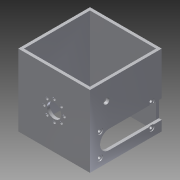
# Autodesk Inventor part: 06
Saved by Autodesk Inventor 2013 (Build 170138000, 138)
## iProperties
Created: 2014-02-01
Material: アルミニウム 6061
Document SubType Name: Modeling
Designer: andou
Density: 1 g/cm^3
Mass: 16.8573 g
Surface Area: 190.608 cm^2
Volume: 16.8573 cm^3
Part Number: 06
Author: andou
Title: Parallel_Case
Autodesk Inventor part; units mm, degrees
ref_plane "YZ Plane" through (0, 0, 0) normal (1, 0, 0) x (0, 1, 0)
ref_plane "XZ Plane" through (0, 0, 0) normal (0, 1, 0) x (-1, 0, 0)
ref_plane "XY Plane" through (0, 0, 0) normal (0, 0, 1) x (1, 0, 0)
sketch "スケッチ1" plane through (0, 0, 0) normal (0, 0, 1) x (1, 0, 0)
  line L0 (-25, 25) -> (25, 25)
  line L1 (25, 25) -> (25, -25)
  line L2 (25, -25) -> (-25, -25)
  line L3 (-25, -25) -> (-25, 25)
  line L4 (-23, 23) -> (23, 23)
  line L5 (23, 23) -> (23, -23)
  line L6 (23, -23) -> (-23, -23)
  line L7 (-23, -23) -> (-23, 23)
  point P0 (0, 0)
  dimension "d0" = 50
  dimension "d1" = 50
  dimension "d4" = 25
  dimension "d5" = 25
  dimension "d6" = 46
  dimension "d7" = 2
  dimension "d8" = 46
  dimension "d9" = 2
  constraints: 16 end point, 4 parallel, 2 horizontal, 2 perpendicular
  measures "d0" distance of L0.start L0.end
  measures "d1" distance of L2.end L0.start
  measures "d4" distance from line of L0 point (0, 0)
  measures "d5" distance from line of L3 point (0, 0)
  measures "d6" distance between parallel lines of L5 L7
  measures "d7" distance between parallel lines of L3 L7
  measures "d8" distance between parallel lines of L4 L6
  measures "d9" distance between parallel lines of L2 L6
extrude "押し出し1" add sketch "スケッチ1" along normal blind 50
sketch "スケッチ11" plane through (25, -25, 0) normal (1, 0, 0) x (0, 0, -1)
  circle A0 centre (-13.5, 13.5) radius 1.5
  circle A1 centre (-37.5, 11.5) radius 1.5
  line L0 (0, 50) -> (0, 0) projected
  line L1 (0, 50) -> (-50, 50) projected
  point P0 (0, 25)
  point P1 (-50, 43)
  dimension "d109" = 3
  dimension "d128" = 2
  dimension "d237" = 36.5
  dimension "d304" = 24
  dimension "d305" = 13.5
  constraints: 2 centre point, 1 equal radius
  measures "d109" diameter of A0
  measures "d128" vertical distance of A1.centre A0.centre
  measures "d237" distance from line of L1 A0.centre
  measures "d304" horizontal distance of A0.centre A1.centre
  measures "d305" distance from line of L0 A0.centre
hole "穴6" at (25, -13.5, 37.5) at (25, -11.5, 13.5) direction (-1, 0, 0) diameter 4 end through all
sketch "スケッチ19" plane through (-25, -25, 0) normal (0, -1, 0) x (1, 0, 0)
  line L0 (50, 50) -> (0, 50) projected
  line L1 (0, 0) -> (0, 50) projected
  circle A0 centre (25, 25) radius 5
  point P0 (25, 0)
  dimension "d306" = 25
  dimension "d307" = 25
  dimension "d308" = 10
  constraints: 1 centre point
  measures "d306" distance from line of L0 A0.centre
  measures "d307" distance from line of L1 A0.centre
  measures "d308" diameter of A0
hole "穴18" at (0, -25, 25) direction (0, 1, 0) diameter 10 depth 2 tip angle 118
sketch "スケッチ20" plane through (-25, -25, 0) normal (0, -1, 0) x (1, 0, 0)
  circle A0 centre (25, 25) radius 5 projected
  line L0 (50, 0) -> (50, 50) projected
  circle A1 centre (25, 32) radius 1
  point P0 (25, 0)
  dimension "d316" = 7
  dimension "d317" = 25
  dimension "d318" = 2
  constraints: 1 centre point
  measures "d316" distance of A1.centre A0.centre
  measures "d317" distance from line of L0 A1.centre
  measures "d318" diameter of A1
hole "穴19" at (0, -25, 32) direction (0, 1, 0) diameter 2 depth 2 tip angle 118
pattern_circular "円形状パターン1" count 8 over 360 about axis through (0, -24, 25) along (0, -1, 0) of "穴19"
sketch "スケッチ21" plane through (25, -25, 0) normal (1, 0, 0) x (0, 0, -1)
  circle A0 centre (-13.5, 13.5) radius 2 projected
  line L0 (0, 50) -> (0, 0) projected
  line L1 (0, 50) -> (-50, 50) projected
  line L2 (-20, 50) -> (-7, 50)
  line L3 (-7, 50) -> (-7, 13.5)
  line L4 (-20, 13.5) -> (-20, 50)
  arc A1 (-20, 13.5) -> (-7, 13.5) centre (-13.5, 13.5) ccw
  point P0 (0, 25)
  dimension "d331" = 13
  dimension "d332" = 6.5
  dimension "d333" = 36.5
  dimension "d334" = 6.5
  dimension "d335" = 13.5
  constraints: 6 end point, 2 point on circle, 1 centre point, 1 horizontal, 1 parallel, 1 perpendicular, 1 point on line
  measures "d331" distance between parallel lines of L4 L3
  measures "d332" distance from line of L3 A0.centre
  measures "d333" distance from line of L1 A1.centre
  measures "d334" radius of A1
  measures "d335" distance from line of L0 A1.centre
extrude "押し出し8" cut sketch "スケッチ21" against normal blind 2
sketch "スケッチ22" plane through (25, -25, 0) normal (1, 0, 0) x (0, 0, -1)
  arc A0 (-20, 13.5) -> (-7, 13.5) centre (-13.5, 13.5) ccw projected
  circle A1 centre (-21.5, 43) radius 1
  circle A2 centre (-21.5, 7) radius 1
  circle A3 centre (-5.5, 43) radius 1
  circle A4 centre (-5.5, 7) radius 1
  circle A5 centre (-13.5, 13.5) radius 2 projected
  point P0 (0, 25)
  dimension "d338" = 16
  dimension "d340" = 16
  dimension "d341" = 8
  dimension "d342" = 8
  dimension "d343" = 2
  dimension "d346" = 36
  dimension "d347" = 36
  dimension "d355" = 6.5
  dimension "d356" = 6.5
  constraints: 4 centre point, 3 equal radius
  measures "d338" distance of A1.centre A3.centre
  measures "d340" distance of A4.centre A2.centre
  measures "d341" horizontal distance of A4.centre A0.centre
  measures "d342" horizontal distance of A0.centre A3.centre
  measures "d343" diameter of A3
  measures "d346" distance of A3.centre A4.centre
  measures "d347" distance of A1.centre A2.centre
  measures "d355" vertical distance of A0.centre A4.centre
  measures "d356" vertical distance of A0.centre A2.centre
hole "穴20" at (25, 18, 21.5) at (25, 18, 5.5) at (25, -18, 5.5) at (25, -18, 21.5) direction (-1, 0, 0) diameter 2 depth 2 tip angle 118 counterbore diameter 4 counterbore depth 0.5
